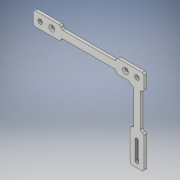
# Autodesk Inventor part: Power Supply Wall Mount v2
Saved by Autodesk Inventor 2019 (Build 230136000, 136)
## iProperties
Created: 2022-03-26
Part Number: Power Supply Wall Mount v2
Material: Generic
Document SubType Name: Modeling
Designer: Lix
Density: 1 g/cm^3
Appearance: Default
Author: Lix
Autodesk Inventor part; units mm, degrees
ref_plane "YZ Plane" through (0, 0, 0) normal (1, 0, 0) x (0, 1, 0)
ref_plane "XZ Plane" through (0, 0, 0) normal (0, 1, 0) x (-1, 0, 0)
ref_plane "XY Plane" through (0, 0, 0) normal (0, 0, 1) x (1, 0, 0)
sketch "Sketch1" plane through (0, 0, 0) normal (0, 0, 1) x (1, 0, 0)
  line L0 (-60, 7.5) -> (60, 7.5)
  line L1 (60, 7.5) -> (60, -7.5)
  line L2 (60, -7.5) -> (-60, -7.5)
  line L3 (-60, -7.5) -> (-60, 7.5)
  line L4 (-60, 7.5) -> (60, -7.5) construction
  line L5 (60, 7.5) -> (-60, -7.5) construction
  circle A0 centre (-52.5, 0) radius 2.5
  circle A1 centre (52.5, 0) radius 2.5
  line L6 (60, -7.5) -> (45, -7.5)
  line L7 (45, -7.5) -> (45, -85)
  line L8 (45, -85) -> (60, -85)
  line L9 (60, -85) -> (60, -7.5)
  circle A2 centre (52.5, -70) radius 2.5 construction
  line L10 (52.5, -79.005) -> (52.5, -59.005) construction
  line L11 (54.5, -79.005) -> (54.5, -59.005)
  line L12 (50.5, -59.005) -> (50.5, -79.005)
  arc A3 (50.5, -79.005) -> (54.5, -79.005) centre (52.5, -79.005) ccw
  arc A4 (54.5, -59.005) -> (50.5, -59.005) centre (52.5, -59.005) ccw
  point P0 (0, 0)
  point P1 (-60, 0)
  point P2 (60, 0)
  point P3 (52.5, -69.005)
  dimension "d0" = 120
  dimension "d1" = 15
  dimension "d2" = 5
  dimension "d3" = 7.5
  dimension "d4" = 7.5
  dimension "d21" = 15
  dimension "d23" = 15
  dimension "d24" = 70
  dimension "d25" = 4
  dimension "d26" = 20
  constraints: 28 end point, 5 centre point, 5 midpoint, 5 parallel, 4 point on circle, 4 tangent, 2 equal radius, 2 horizontal, 2 horizontal alignment, 2 perpendicular, 2 vertical alignment, 1 vertical
  measures "d0" distance of L1.end L2.end
  measures "d1" distance of L0.end L1.end
  measures "d2" diameter of A0
  measures "d3" distance from line of L3 A0.centre
  measures "d4" distance from line of L1 A1.centre
  measures "d21" distance of L8.end L7.end
  measures "d23" distance from line of A2.centre L8
  measures "d24" distance of A2.centre A1.centre
  measures "d25" diameter of A4
  measures "d26" distance of L11.start L11.end
extrude "Extrusion1" add sketch "Sketch1" along normal blind 3
sketch "Sketch2" plane through (0, 0, 3) normal (0, 0, 1) x (1, 0, 0)
  line L0 (-40, 0) -> (40, 0) construction
  point P0 (0, 0)
  point P1 (0, 0)
  dimension "d7" = 80
  constraints: 2 end point, 2 horizontal alignment, 1 coincident, 1 horizontal, 1 midpoint
  measures "d7" distance of L0.start L0.end
hole "Hole1" at (-40, 0, 3) at (40, 0, 3) direction (0, 0, -1) diameter 3.3 depth 36.25 countersink diameter 6.5 countersink angle 90
sketch "Sketch3" plane through (0, 0, 3) normal (0, 0, 1) x (1, 0, 0)
  line L0 (-30, 7.5) -> (30, 7.5)
  line L1 (30, 7.5) -> (30, 4)
  line L2 (30, 4) -> (-30, 4)
  line L3 (-30, 4) -> (-30, 7.5)
  circle A0 centre (-40, 0) radius 1.65 projected
  circle A1 centre (40, 0) radius 1.65 projected
  line L4 (60, 7.5) -> (-60, 7.5) projected
  point P0 (0, 0)
  dimension "d16" = 10
  dimension "d17" = 10
  dimension "d18" = 4
  constraints: 8 end point, 2 parallel, 1 collinear, 1 horizontal, 1 perpendicular
  measures "d16" distance from line of L3 A0.centre
  measures "d17" distance from line of A1.centre L1
  measures "d18" distance from line of point (0, 0) L2
extrude "Extrusion2" cut sketch "Sketch3" against normal blind 3 contours L0 L1 L2 L3
ref_plane "Work Plane1" through (-60, 0, 3) normal (0, 1, 0) x (1, 0, 0)
mirror "Mirror1" about plane through (-60, 0, 3) normal (0, 1, 0) of "Extrusion2"
fillet "Fillet1" radius 2 14 edges at (-60, 7.5, 1.5) (-60, -7.5, 1.5) (60, 7.5, 1.5) (-30, 7.5, 1.5) (-30, 4, 1.5) (-30, -4, 1.5) (-30, -7.5, 1.5) (30, 7.5, 1.5) (30, 4, 1.5) (30, -7.5, 1.5) (30, -4, 1.5) (45, -7.5, 1.5) (45, -85, 1.5) (60, -85, 1.5)
sketch "Sketch4" plane through (0, 0, 3) normal (0, 0, 1) x (1, 0, 0)
  line L0 (45, -49.005) -> (49, -49.005)
  line L1 (49, -49.005) -> (49, -10)
  line L2 (49, -10) -> (45, -10)
  line L3 (45, -10) -> (45, -49.005)
  line L4 (45, -9.5) -> (45, -83) projected
  arc A0 (54.5, -59.005) -> (50.5, -59.005) centre (52.5, -59.005) ccw projected
  circle A1 centre (40, 0) radius 1.65 projected
  point P0 (0, 0)
  dimension "d27" = 4
  dimension "d28" = 10
  dimension "d29" = 10
  constraints: 8 end point, 2 parallel, 1 collinear, 1 horizontal, 1 perpendicular
  measures "d27" distance between parallel lines of L1 L4
  measures "d28" distance from line of L0 A0.centre
  measures "d29" distance from line of L2 A1.centre
extrude "Extrusion3" cut sketch "Sketch4" against normal blind 10 contours L3 L2 L1 L0
ref_plane "Work Plane2" through (52.5, -83, 0) normal (-1, 0, 0) x (0, 0, 1)
mirror "Mirror2" about plane through (52.5, -83, 0) normal (-1, 0, 0) of "Extrusion3"
fillet "Fillet2" radius 2 8 edges at (60, -49.005, 1.5) (56, -49.005, 1.5) (45, -49.005, 1.5) (49, -49.005, 1.5) (56, -10, 1.5) (60, -10, 1.5) (45, -10, 1.5) (49, -10, 1.5)
equation "\"d4\" = d3"
equation "\"d17\" = d16"
body "Solid1"
